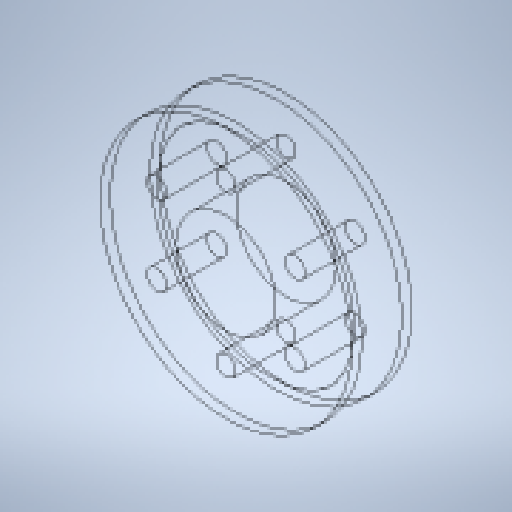
# Autodesk Inventor part: Pulley
Saved by Autodesk Inventor 2023.2 (Build 272271000, 271)
## iProperties
Created: 2023-11-16
Part Number: Pulley
Material: Nylon 6/6
Document SubType Name: Modeling
Designer: Nathan Cai
Density: 1.13 g/cm^3
Appearance: Rubber - Blue
Author: Nathan Cai
Autodesk Inventor part; units mm, degrees
ref_plane "YZ Plane" through (0, 0, 0) normal (1, 0, 0) x (0, 1, 0)
ref_plane "XZ Plane" through (0, 0, 0) normal (0, 1, 0) x (-1, 0, 0)
ref_plane "XY Plane" through (0, 0, 0) normal (0, 0, 1) x (1, 0, 0)
sketch "Sketch1" plane through (0, 0, 0) normal (1, 0, 0) x (0, 1, 0)
  line L0 (-20, 4.7625) -> (20, 4.7625)
  line L1 (20, 4.7625) -> (20, -4.7625)
  line L2 (20, -4.7625) -> (-20, -4.7625)
  line L3 (-20, -4.7625) -> (-20, 4.7625)
  line L4 (-20, 4.7625) -> (20, -4.7625) construction
  line L5 (20, 4.7625) -> (-20, -4.7625) construction
  circle A0 centre (20, 0) radius 3.175
  circle A1 centre (-20, 0) radius 3.175
  line L6 (-7.9375, 4.7625) -> (7.9375, 4.7625)
  line L7 (7.9375, 4.7625) -> (7.9375, -4.7625)
  line L8 (7.9375, -4.7625) -> (-7.9375, -4.7625)
  line L9 (-7.9375, -4.7625) -> (-7.9375, 4.7625)
  line L10 (-7.9375, 4.7625) -> (7.9375, -4.7625) construction
  line L11 (7.9375, 4.7625) -> (-7.9375, -4.7625) construction
  line L12 (0, 4.7625) -> (0, -4.7625) construction
  point P0 (0, 0)
  point P1 (20, -3.175)
  point P2 (20, 3.175)
  dimension "d0" = 9.525
  dimension "d1" = 40
  dimension "d2" = 6.35
  dimension "d3" = 6.35
  dimension "d4" = 15.875
  constraints: 26 end point, 8 midpoint, 4 parallel, 2 centre point, 2 horizontal, 2 perpendicular, 1 point on line
  measures "d0" distance of L0.end L1.end
  measures "d1" distance between parallel lines of L3 L1
  measures "d2" diameter of A0
  measures "d3" diameter of A1
  measures "d4" distance of L7.end L8.end
revolve "Revolution1" add sketch "Sketch1" angle 360 about axis through (0, 0, 4.7625) along (0, 0, -1) contours L0 L1 A0 L2 L7
sketch "Sketch2" plane through (0, 0, 4.7625) normal (0, 0, 1) x (1, 0, 0)
  circle A0 centre (0, 0) radius 12.7 construction
  circle A1 centre (0, 12.7) radius 1.5875
  line L0 (0, 12.7) -> (0, 0) construction
  circle A2 centre (-10.9985, 6.35) radius 1.5875
  circle A3 centre (-10.9985, -6.35) radius 1.5875
  circle A4 centre (0, -12.7) radius 1.5875
  circle A5 centre (10.9985, -6.35) radius 1.5875
  circle A6 centre (10.9985, 6.35) radius 1.5875
  dimension "d6" = 25.4
  dimension "d7" = 3.175
  dimension "d10" = 360
  constraints: 6 centre point, 2 end point, 1 coincident, 1 vertical, 1 vertical alignment, 15 other
  measures "d7" diameter of A1
extrude "Extrusion1" cut sketch "Sketch2" against normal through all
sketch "Sketch3" plane through (0, 0, 4.7625) normal (0, 0, 1) x (1, 0, 0)
  circle A0 centre (0, 0) radius 11
  dimension "d14" = 22
  constraints: 1 centre point, 1 coincident
  measures "d14" diameter of A0
extrude "Extrusion2" cut sketch "Sketch3" against normal blind 3.175
chamfer "Chamfer1" distance 3.175 angle 45 1 edges at (-11, 0, 4.7625)
body "Solid1"
